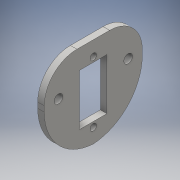
# Autodesk Inventor part: new_micro_servo_mount
Saved by Autodesk Inventor 2016 (Build 200138000, 138)
## iProperties
Created: 2024-02-03
Part Number: new_micro_servo_mount
Material: Generic
Document SubType Name: Modeling
Designer: Dell
Density: 1 g/cm^3
Appearance: Default
Author: Dell
Autodesk Inventor part; units mm, degrees
ref_plane "YZ Plane" through (0, 0, 0) normal (1, 0, 0) x (0, 1, 0)
ref_plane "XZ Plane" through (0, 0, 0) normal (0, 1, 0) x (-1, 0, 0)
ref_plane "XY Plane" through (0, 0, 0) normal (0, 0, 1) x (1, 0, 0)
sketch "Sketch1" plane through (0, 0, 0) normal (1, 0, 0) x (0, 1, 0)
  line L0 (10, 0) -> (25, 0)
  line L1 (40, -15) -> (40, -17.5)
  line L2 (-5, -17.5) -> (-5, -15)
  line L3 (23.75, -9) -> (11.25, -9)
  line L4 (11.25, -9) -> (11.25, -32.5)
  line L5 (11.25, -32.5) -> (23.75, -32.5)
  line L6 (23.75, -32.5) -> (23.75, -9)
  circle A0 centre (17.5, -6.75) radius 1.5
  circle A1 centre (17.5, -34.75) radius 1.5
  arc A2 (10, 0) -> (-5, -15) centre (10, -15) ccw
  arc A3 (40, -15) -> (25, 0) centre (25, -15) ccw
  arc A4 (-5, -17.5) -> (17.5, -41.4531) centre (19, -17.5) ccw
  arc A5 (17.5, -41.4531) -> (40, -17.5) centre (16, -17.5) ccw
  point P0 (40, -41.5)
  point P1 (40, 0)
  point P2 (-5, -41.5)
  dimension "d0" = 41.5
  dimension "d1" = 45
  dimension "d3" = 12.5
  dimension "d4" = 23.5
  dimension "d5" = 16.25
  dimension "d6" = 3
  dimension "d7" = 2.25
  dimension "d8" = 2.25
  dimension "d30" = 3
  dimension "d31" = 6.75
  dimension "d32" = 22.5
  dimension "d33" = 22.5
  dimension "d62" = 15
  dimension "d63" = 24
  constraints: 14 end point, 8 point on circle, 6 centre point, 6 tangent, 4 point on line, 3 parallel, 2 equal radius, 2 horizontal, 2 perpendicular
  measures "d0" distance of point (40, 0) point (40, -41.5)
  measures "d1" distance of point (40, -41.5) point (-5, -41.5)
  measures "d3" distance of L4.end L5.end
  measures "d4" distance of L3.end L4.end
  measures "d5" distance between parallel lines of L2 L4
  measures "d6" diameter of A0
  measures "d7" distance from line of L3 A0.centre
  measures "d8" distance from line of L5 A1.centre
  measures "d30" diameter of A1
  measures "d31" distance from line of A0.centre L0
  measures "d32" distance from line of L2 A0.centre
  measures "d33" distance from line of A1.centre L2
  measures "d62" radius of A2
  measures "d63" radius of A4
extrude "Extrusion1" add sketch "Sketch1" along normal blind 3
sketch "Sketch11" plane through (3, 0, 0) normal (1, 0, 0) x (0, 0, -1)
  circle A0 centre (15.5, 1.5) radius 2
  circle A1 centre (15.5, 33.5) radius 2
  line L0 (0, 25) -> (0, 0) projected
  circle A2 centre (6.75, 17.5) radius 1.5 projected
  point P0 (0, 40)
  dimension "d55" = 15.5
  dimension "d56" = 16
  dimension "d57" = 4
  dimension "d58" = 4
  dimension "d60" = 15.5
  dimension "d61" = 16
  constraints: 2 centre point
  measures "d55" distance from line of A1.centre L0
  measures "d56" vertical distance of A2.centre A1.centre
  measures "d57" diameter of A1
  measures "d58" diameter of A0
  measures "d60" distance from line of L0 A0.centre
  measures "d61" vertical distance of A2.centre A0.centre
extrude "Extrusion11" cut sketch "Sketch11" against normal through all contours A0 | A1
body "Solid1"
